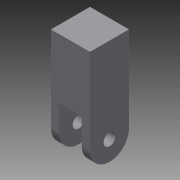
# Autodesk Inventor part: spoke
Saved by Autodesk Inventor 2014 SP2 (Build 180246200, 246)
## iProperties
Created: 2016-12-02
Part Number: spoke
Material: Generic
Document SubType Name: Modeling
Designer: Justin B
Density: 1 g/cm^3
Appearance: Default
Author: Justin B
Autodesk Inventor part; units mm, degrees
ref_plane "YZ Plane" through (0, 0, 0) normal (1, 0, 0) x (0, 1, 0)
ref_plane "XZ Plane" through (0, 0, 0) normal (0, 1, 0) x (-1, 0, 0)
ref_plane "XY Plane" through (0, 0, 0) normal (0, 0, 1) x (1, 0, 0)
sketch "Sketch1" plane through (0, 0, 0) normal (0, 1, 0) x (-1, 0, 0)
  line L0 (-7.5, 0) -> (7.5, 0)
  line L1 (7.5, 0) -> (7.5, -30)
  line L2 (7.5, -30) -> (13, -30)
  line L3 (13, -30) -> (13, 40)
  line L4 (13, 40) -> (-13, 40)
  line L5 (-13, 40) -> (-13, -30)
  line L6 (-13, -30) -> (-7.5, -30)
  line L7 (-7.5, -30) -> (-7.5, 0)
  line L8 (0, 0) -> (0, 40) construction
  line L9 (-11, 8) -> (11, 8) construction
  point P0 (0, 8)
  dimension "d0" = 22
  dimension "d1" = 30
  dimension "d2" = 15
  dimension "d3" = 8
  dimension "d8" = 26
  dimension "d9" = 40
  constraints: 20 end point, 6 parallel, 4 midpoint, 3 perpendicular, 1 horizontal, 1 vertical, 1 vertical alignment, 2 other
  measures "d0" distance of L9.start L9.end
  measures "d1" distance of L0.end L1.end
  measures "d2" distance of L0.start L0.end
  measures "d3" distance from line of L0 point (0, 8)
  measures "d8" distance of L3.end L4.end
  measures "d9" distance between parallel lines of L4 L0
extrude "Extrusion1" add sketch "Sketch1" along normal blind 26
sketch "Sketch2" plane through (13, 0, 40) normal (1, 0, 0) x (0, 0, -1)
  line L0 (70, 0) -> (70, 26) projected
  circle A0 centre (57, 13) radius 4
  point P0 (40, 0)
  point P1 (70, 13)
  dimension "d10" = 8
  dimension "d11" = 13
  constraints: 1 centre point, 1 horizontal alignment, 1 midpoint
  measures "d10" diameter of A0
  measures "d11" distance from line of L0 A0.centre
extrude "Extrusion2" cut sketch "Sketch2" against normal up to surface (26 mm away)
fillet "Fillet1" radius 13 4 edges at (-10.25, 26, -30) (10.25, 26, -30) (-10.25, 0, -30) (10.25, 0, -30)
sketch "Sketch3" plane through (-13, 0, 40) normal (0, 0, 1) x (1, 0, 0)
  line L0 (0, 0) -> (26, 0) projected
  line L1 (26, 0) -> (26, 26) projected
  circle A0 centre (13, 13) radius 11
  point P0 (13, 0)
  point P1 (26, 13)
  point P2 (13, 0)
  dimension "d15" = 22
  constraints: 2 midpoint, 1 centre point, 1 horizontal alignment, 1 vertical alignment
  measures "d15" diameter of A0
extrude "Extrusion3" cut sketch "Sketch3" against normal blind 35
body "Solid1"
